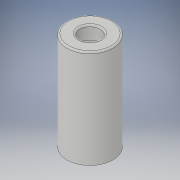
# Autodesk Inventor part: peça encaixe telhado
Saved by Autodesk Inventor 2019.4 (Build 234330000, 330)
## iProperties
Created: 2020-08-29
Part Number: peça encaixe telhado
Material: Genérico
Document SubType Name: Modeling
Designer: Lattes
Density: 1 g/cm^3
Appearance: Padrão
Author: Lattes
## iProperties of the stored document _3DPrint.ipt
Created: 2020-08-29
Part Number: _3DPrint
Material: Genérico
Document SubType Name: Modeling
Designer: Lattes
Density: 1 g/cm^3
Appearance: Padrão
Author: Lattes
Autodesk Inventor part; units mm, degrees
ref_plane "YZ Plane" through (0, 0, 0) normal (1, 0, 0) x (0, 1, 0)
ref_plane "XZ Plane" through (0, 0, 0) normal (0, 1, 0) x (-1, 0, 0)
ref_plane "XY Plane" through (0, 0, 0) normal (0, 0, 1) x (1, 0, 0)
sketch "Esboço1" plane through (0, 0, 0) normal (0, 1, 0) x (-1, 0, 0)
  circle A0 centre (0, 0) radius 3.31
  circle A1 centre (0, 0) radius 14
  dimension "d2" = 6.62
  dimension "d3" = 28
  constraints: 2 centre point, 1 coincident
  measures "d2" diameter of A0
  measures "d3" diameter of A1
extrude "Extrusão1" add sketch "Esboço1" along normal blind 60
sketch "Esboço2" plane through (0, 60, 0) normal (0, 1, 0) x (1, 0, 0)
  circle A0 centre (0, 0) radius 6.25
  dimension "d7" = 12.5
  constraints: 1 centre point
  measures "d7" diameter of A0
extrude "Extrusão2" cut sketch "Esboço2" against normal blind 9
sketch "Esboço3" plane through (0, 0, 0) normal (0, -1, 0) x (1, 0, 0)
  circle A0 centre (0, 0) radius 3.31
  constraints: 1 centre point, 1 coincident
extrude "Extrusão3" add sketch "Esboço3" against normal blind 30
fillet "Arredondamento1" radius 1 5 edges at (14, 60, 0) (-6.25, 60, 0) (-6.25, 51, 0) (3.31, 51, 0) (3.31, 30, 0)
